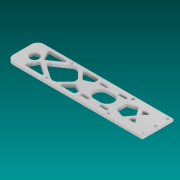
# Autodesk Inventor part: bovenarm - links
Saved by Autodesk Inventor 2020 (Build 240168000, 168)
## iProperties
Created: 2020-05-18
Part Number: bovenarm - links
Material: Aluminum 6061
Document SubType Name: Modeling
Designer: stefa
Density: 2.7 g/cm^3
Appearance: Aluminum - Polished
Mass: 81.5544 g
Surface Area: 207.298 cm^2
Volume: 30.2053 cm^3
Author: stefa
Autodesk Inventor part; units mm, degrees
ref_plane "YZ Plane" through (0, 0, 0) normal (1, 0, 0) x (0, 1, 0)
ref_plane "XZ Plane" through (0, 0, 0) normal (0, 1, 0) x (-1, 0, 0)
ref_plane "XY Plane" through (0, 0, 0) normal (0, 0, 1) x (1, 0, 0)
sketch "Sketch1" plane through (0, 0, 0) normal (0, 1, 0) x (-1, 0, 0)
  line L0 (0, 0) -> (220, 0)
  line L1 (220, 0) -> (220, -50)
  line L2 (220, -50) -> (0, -50)
  line L3 (0, -50) -> (0, 0)
  circle A0 centre (200, -25) radius 7
  line L4 (92.355, -25) -> (82.355, -25) construction
  line L5 (92.355, -13.9) -> (82.355, -13.9)
  line L6 (82.355, -36.1) -> (92.355, -36.1)
  arc A1 (92.355, -36.1) -> (92.355, -13.9) centre (92.355, -25) ccw
  arc A2 (82.355, -13.9) -> (82.355, -36.1) centre (82.355, -25) ccw
  line L7 (107.855, -40.5) -> (97.855, -40.5) construction
  line L8 (107.855, -38.95) -> (97.855, -38.95)
  line L9 (97.855, -42.05) -> (107.855, -42.05)
  arc A3 (107.855, -42.05) -> (107.855, -38.95) centre (107.855, -40.5) ccw
  arc A4 (97.855, -38.95) -> (97.855, -42.05) centre (97.855, -40.5) ccw
  line L10 (66.855, -42.05) -> (76.855, -42.05)
  arc A5 (76.855, -42.05) -> (76.855, -38.95) centre (76.855, -40.5) ccw
  line L11 (76.855, -40.5) -> (66.855, -40.5) construction
  line L12 (76.855, -38.95) -> (66.855, -38.95)
  arc A6 (66.855, -38.95) -> (66.855, -42.05) centre (66.855, -40.5) ccw
  line L13 (97.855, -11.05) -> (107.855, -11.05)
  arc A7 (107.855, -11.05) -> (107.855, -7.95) centre (107.855, -9.5) ccw
  line L14 (107.855, -9.5) -> (97.855, -9.5) construction
  line L15 (107.855, -7.95) -> (97.855, -7.95)
  arc A8 (97.855, -7.95) -> (97.855, -11.05) centre (97.855, -9.5) ccw
  line L16 (66.855, -11.05) -> (76.855, -11.05)
  arc A9 (76.855, -11.05) -> (76.855, -7.95) centre (76.855, -9.5) ccw
  line L17 (76.855, -9.5) -> (66.855, -9.5) construction
  line L18 (76.855, -7.95) -> (66.855, -7.95)
  arc A10 (66.855, -7.95) -> (66.855, -11.05) centre (66.855, -9.5) ccw
  circle A11 centre (160, -5) radius 2
  circle A12 centre (160, -45) radius 2
  circle A13 centre (60, -5) radius 2
  circle A14 centre (60, -45) radius 2
  circle A15 centre (4, -25) radius 2
  circle A16 centre (4, -45) radius 2
  circle A17 centre (4, -5) radius 2
  point P0 (87.355, -25)
  point P1 (102.855, -40.5)
  point P2 (71.855, -40.5)
  point P3 (102.855, -9.5)
  point P4 (71.855, -9.5)
  point P5 (0, -25)
  dimension "d0" = 220
  dimension "d1" = 50
  dimension "d16" = 14
  dimension "d18" = 25
  dimension "d24" = 22.2
  dimension "d25" = 3.1
  dimension "d26" = 10
  dimension "d27" = 10
  dimension "d28" = 112.645
  dimension "d29" = 25
  dimension "d31" = 15.5
  dimension "d32" = 15.5
  dimension "d35" = 31
  dimension "d38" = 31
  dimension "d42" = 4
  dimension "d44" = 5
  dimension "d47" = 40
  dimension "d50" = 100
  dimension "d53" = 4
  dimension "d54" = 4
  dimension "d55" = 20
  dimension "d56" = 20
  dimension "d106" = 200
  dimension "d107" = 160
  constraints: 48 end point, 20 point on circle, 18 centre point, 8 tangent, 5 parallel, 4 horizontal, 3 midpoint, 2 equal radius, 2 vertical, 2 vertical alignment, 1 horizontal alignment, 1 perpendicular, 42 other
  measures "d0" distance of L1.end L2.end
  measures "d1" distance of L0.end L1.end
  measures "d16" diameter of A0
  measures "d18" distance from line of L0 A0.centre
  measures "d24" diameter of A2
  measures "d25" diameter of A4
  measures "d26" distance of L9.start L9.end
  measures "d27" distance of L6.start L6.end
  measures "d28" distance of A0.centre point (87.355, -25)
  measures "d29" distance from line of L0 point (87.355, -25)
  measures "d31" horizontal distance of point (87.355, -25) point (102.855, -40.5)
  measures "d32" horizontal distance of point (102.855, -40.5) point (87.355, -25)
  measures "d35" distance of L9.start L10.start
  measures "d38" distance of L9.start L13.start
  measures "d42" diameter of A11
  measures "d44" distance from line of L0 A11.centre
  measures "d47" distance of A11.centre A12.centre
  measures "d50" distance of A11.centre A13.centre
  measures "d53" diameter of A15
  measures "d54" distance from line of L3 A15.centre
  measures "d55" distance of A17.centre A15.centre
  measures "d56" distance of A16.centre A15.centre
  measures "d106" distance from line of L3 A0.centre
  measures "d107" distance from line of L3 A11.centre
extrude "Extrusion1" add sketch "Sketch1" along normal blind 4
fillet "Fillet1" radius 10 2 edges at (-220, 2, 0) (-220, 2, -50)
sketch "Sketch4" plane through (0, 4, 0) normal (0, 1, 0) x (1, 0, 0)
  arc A0 (-92.355, 36.1) -> (-92.355, 13.9) centre (-92.355, 25) ccw projected
  line L0 (-92.355, 36.1) -> (-82.355, 36.1) projected
  arc A1 (-82.355, 13.9) -> (-82.355, 36.1) centre (-82.355, 25) ccw projected
  line L1 (-82.355, 13.9) -> (-92.355, 13.9) projected
  line L2 (-76.855, 11.05) -> (-66.855, 11.05) projected
  arc A2 (-66.855, 7.95) -> (-66.855, 11.05) centre (-66.855, 9.5) ccw projected
  line L3 (-66.855, 7.95) -> (-76.855, 7.95) projected
  arc A3 (-76.855, 11.05) -> (-76.855, 7.95) centre (-76.855, 9.5) ccw projected
  line L4 (-107.855, 11.05) -> (-97.855, 11.05) projected
  arc A4 (-97.855, 7.95) -> (-97.855, 11.05) centre (-97.855, 9.5) ccw projected
  line L5 (-97.855, 7.95) -> (-107.855, 7.95) projected
  arc A5 (-107.855, 11.05) -> (-107.855, 7.95) centre (-107.855, 9.5) ccw projected
  line L6 (-97.855, 38.95) -> (-107.855, 38.95) projected
  arc A6 (-107.855, 42.05) -> (-107.855, 38.95) centre (-107.855, 40.5) ccw projected
  line L7 (-107.855, 42.05) -> (-97.855, 42.05) projected
  arc A7 (-97.855, 38.95) -> (-97.855, 42.05) centre (-97.855, 40.5) ccw projected
  arc A8 (-76.855, 42.05) -> (-76.855, 38.95) centre (-76.855, 40.5) ccw projected
  line L8 (-76.855, 42.05) -> (-66.855, 42.05) projected
  arc A9 (-66.855, 38.95) -> (-66.855, 42.05) centre (-66.855, 40.5) ccw projected
  line L9 (-66.855, 38.95) -> (-76.855, 38.95) projected
  circle A10 centre (-200, 25) radius 7 projected
  circle A11 centre (-160, 5) radius 2 projected
  circle A12 centre (-160, 45) radius 2 projected
  circle A13 centre (-60, 5) radius 2 projected
  circle A14 centre (-60, 45) radius 2 projected
  circle A15 centre (-4, 25) radius 2 projected
  circle A16 centre (-4, 45) radius 2 projected
  circle A17 centre (-4, 5) radius 2 projected
  arc A18 (-210, 50) -> (-220, 40) centre (-210, 40) ccw projected
  line L10 (-210, 0) -> (0, 0) projected
  line L11 (0, 0) -> (0, 50) projected
  line L12 (0, 50) -> (-210, 50) projected
  line L13 (-200, 25) -> (-4, 25) construction
  line L14 (-198, 5) -> (-163, 5)
  line L15 (-163, 5) -> (-188, 22.3205)
  line L16 (-188, 22.3205) -> (-198, 5)
  line L17 (-142, 5) -> (-115, 5)
  line L18 (-115, 5) -> (-115, 13)
  line L19 (-115, 13) -> (-128, 19)
  line L20 (-128, 19) -> (-142, 5)
  line L21 (-182, 25) -> (-157, 7.6795)
  line L22 (-132, 25) -> (-182, 25)
  line L23 (-30.9142, 20) -> (-24, 13)
  line L24 (-24, 13) -> (-36, 13)
  line L25 (-36, 13) -> (-30.9142, 20)
  line L26 (-34.3896, 25) -> (-43.7942, 12.0557)
  line L27 (-43.7942, 12.0557) -> (-59.0111, 17)
  line L28 (-59.0111, 17) -> (-59.0111, 33)
  line L29 (-59.0111, 33) -> (-43.7942, 37.9443)
  line L30 (-43.7942, 37.9443) -> (-34.3896, 25)
  line L31 (0, 0) -> (0, 50) projected
  arc A19 (-157, 7.6795) -> (-145.2644, 8.7356) centre (-151.7647, 15.236) ccw
  line L32 (-132, 25) -> (-132, 22)
  line L33 (-132, 22) -> (-145.2644, 8.7356)
  line L34 (-198, 45) -> (-163, 45)
  line L35 (-163, 45) -> (-188, 27.6795)
  line L36 (-188, 27.6795) -> (-198, 45)
  line L37 (-142, 45) -> (-115, 45)
  line L38 (-115, 45) -> (-115, 37)
  line L39 (-115, 37) -> (-128, 31)
  line L40 (-128, 31) -> (-142, 45)
  line L41 (-182, 25) -> (-157, 42.3205)
  line L42 (-30.9142, 30) -> (-24, 37)
  line L43 (-24, 37) -> (-36, 37)
  line L44 (-36, 37) -> (-30.9142, 30)
  line L45 (-34.3896, 25) -> (-43.7942, 37.9443)
  line L46 (-43.7942, 37.9443) -> (-59.0111, 33)
  line L47 (-59.0111, 33) -> (-59.0111, 17)
  line L48 (-59.0111, 17) -> (-43.7942, 12.0557)
  line L49 (-43.7942, 12.0557) -> (-34.3896, 25)
  arc A20 (-145.2644, 41.2644) -> (-157, 42.3205) centre (-151.7647, 34.764) ccw
  line L50 (-132, 28) -> (-145.2644, 41.2644)
  line L51 (-132, 25) -> (-132, 28)
  line L52 (-220, 40) -> (-220, 10) projected
  arc A21 (-220, 10) -> (-210, 0) centre (-210, 10) ccw projected
  point P0 (-48, 25)
  dimension "d66" = 5
  dimension "d67" = 60
  dimension "d70" = 24
  dimension "d71" = 12
  dimension "d72" = 7
  dimension "d73" = 5
  dimension "d74" = 16
  dimension "d75" = 48
  dimension "d79" = 20
  dimension "d80" = 163
  dimension "d81" = 35
  dimension "d82" = 132
  dimension "d85" = 50
  dimension "d86" = 45
  dimension "d87" = 3
  dimension "d88" = 8
  dimension "d89" = 115
  dimension "d92" = 14
  dimension "d93" = 13
  constraints: 78 end point, 18 symmetric about line, 6 parallel, 5 point on line, 4 horizontal, 4 point on circle, 2 centre point, 2 tangent, 1 perpendicular, 1 vertical, 12 other
  measures "d66" distance between parallel lines of L10 L14
  measures "d67" angle of L14 L16
  measures "d70" distance from line of L11 L23.end
  measures "d71" distance of L23.end L24.end
  measures "d72" distance from line of L24 L23.start
  measures "d73" distance from line of L23.start L13
  measures "d74" distance of L27.end L28.end
  measures "d75" distance from line of L11 point (-48, 25)
  measures "d79" distance of L15.end L14.start
  measures "d80" distance from line of L11 L14.end
  measures "d81" distance of L14.start L14.end
  measures "d82" distance from line of L11 L22.start
  measures "d85" distance of L22.start L21.start
  measures "d86" angle of L33 L22
  measures "d87" distance of L22.start L32.end
  measures "d88" distance of L17.end L18.end
  measures "d89" distance from line of L11 L17.end
  measures "d92" distance from line of L17 L19.end
  measures "d93" distance from line of L18 L19.end
extrude "Extrusion2" cut sketch "Sketch4" against normal blind 10 contours L16 L15 L14 | L20 L19 L18 L17 | L22 L32 L33 A19 L21 | L41 A20 L50 L51 L22 | L23 L24 L25 | L26 L27 L28 L29 L30 | L34 L35 L36 | L37 L38 L39 L40 | L44 L43 L42
fillet "Fillet2" radius 2 6 edges at (-198, 2, -45) (-188, 2, -27.6795) (-163, 2, -45) (-188, 2, -22.3205) (-198, 2, -5) (-163, 2, -5)
fillet "Fillet3" radius 8 2 edges at (-132, 2, -28) (-132, 2, -22)
fillet "Fillet4" radius 3 1 edges at (-182, 2, -25)
fillet "Fillet5" radius 2 4 edges at (-142, 2, -45) (-128, 2, -31) (-128, 2, -19) (-142, 2, -5)
fillet "Fillet6" radius 3 4 edges at (-115, 2, -45) (-115, 2, -37) (-115, 2, -13) (-115, 2, -5)
fillet "Fillet7" radius 2 5 edges at (-59.0111, 2, -33) (-59.0111, 2, -17) (-43.7942, 2, -12.0557) (-43.7942, 2, -37.9443) (-34.3896, 2, -25)
fillet "Fillet8" radius 1 6 edges at (-36, 2, -13) (-30.9142, 2, -20) (-24, 2, -13) (-30.9142, 2, -30) (-36, 2, -37) (-24, 2, -37)
equation "\"d18\" = 0.5 * d1"
equation "\"d56\" = d55"
body "Solid1"
